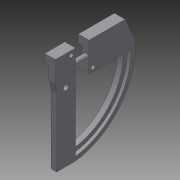
# Autodesk Inventor part: eye_cam_angled_bracket
Saved by Autodesk Inventor 2015 (Build 190159000, 159)
## iProperties
Created: 2015-06-20
Part Number: eye_cam_angled_bracket
Material: Generic
Document SubType Name: Modeling
Designer: Master
Density: 1 g/cm^3
Appearance: Default
Author: Master
Autodesk Inventor part; units mm, degrees
ref_plane "YZ Plane" through (0, 0, 0) normal (1, 0, 0) x (0, 1, 0)
ref_plane "XZ Plane" through (0, 0, 0) normal (0, 1, 0) x (-1, 0, 0)
ref_plane "XY Plane" through (0, 0, 0) normal (0, 0, 1) x (1, 0, 0)
sketch "Sketch1" plane through (0, 0, 0) normal (0, 0, 1) x (1, 0, 0)
  circle A0 centre (0, 0) radius 2
  dimension "d0" = 4
  constraints: 1 centre point, 1 coincident
  measures "d0" diameter of A0
extrude "Extrusion1" add sketch "Sketch1" against normal blind 40
sketch "Sketch2" plane through (0, 0, 0) normal (0, 0, 1) x (1, 0, 0)
  circle A0 centre (0, 0) radius 2 projected
  line L0 (2, -4.5) -> (-3, -4.5)
  line L1 (-3, -4.5) -> (-3, 4.5)
  line L2 (-3, 4.5) -> (2, 4.5)
  line L3 (2, 4.5) -> (2, -4.5)
  dimension "d3" = 3
  dimension "d4" = 9
  dimension "d5" = 4.5
  constraints: 8 end point, 1 tangent
  measures "d3" distance from line of L1 point (0, 0)
  measures "d4" distance between parallel lines of L2 L0
  measures "d5" distance from line of point (0, 0) L0
extrude "Extrusion2" add sketch "Sketch2" along normal blind 6 contours A0 | L3 L0 L1 L2
sketch "Sketch3" plane through (0, 0, 6) normal (0, 0, 1) x (1, 0, 0)
  circle A0 centre (0, 0) radius 2 projected
  line L0 (-3, -4.5) -> (2, -4.5) projected
  line L1 (2, -4.5) -> (2, 4.5) projected
  line L2 (2, 4.5) -> (-3, 4.5) projected
  line L3 (-3, 4.5) -> (-3, -4.5) projected
  line L4 (2, -4.5) -> (2, 4.5) projected
  line L5 (-3, 4.5) -> (2, 4.5)
  line L6 (2, 4.5) -> (2, 3.5)
  line L7 (2, 3.5) -> (-3, 3.5)
  line L8 (-3, 3.5) -> (-3, 4.5)
  point P0 (2, 0)
  dimension "d8" = 1
  constraints: 8 end point, 1 horizontal alignment, 1 point on line
  measures "d8" distance between parallel lines of L2 L7
extrude "Extrusion3" cut sketch "Sketch3" against normal blind 6 contours L7 L3 L2 L1
sketch "Sketch4" plane through (0, 0, -40) normal (0, 0, -1) x (-1, 0, 0)
  circle A0 centre (0, 0) radius 2 projected
extrude "Extrusion4" cut sketch "Sketch4" against normal blind 6
sketch "Sketch5" plane through (0, 0, -34) normal (0, 0, -1) x (-1, 0, 0)
  line L0 (3, 3.5) -> (-2, 3.5) projected
  line L1 (3, -4.5) -> (3, 3.5) projected
  line L2 (-2, 3.5) -> (-2, 0) projected
  line L3 (-2, 0) -> (-2, -4.5) projected
  line L4 (-2, -4.5) -> (3, -4.5) projected
  line L5 (3, 3.5) -> (-2, 3.5)
  line L6 (-2, 3.5) -> (-2, -4.5)
  line L7 (-2, -4.5) -> (3, -4.5)
  line L8 (3, -4.5) -> (3, 3.5)
  point P0 (0, 0)
  constraints: 8 end point
extrude "Extrusion5" add sketch "Sketch5" along normal blind 12
sketch "Sketch6" plane through (-3, -4.5, -34) normal (0, -1, 0) x (1, 0, 0)
  line L0 (5, 0) -> (0, 0) projected
  line L1 (0, 0) -> (0, -12) projected
  line L2 (5, -12) -> (0, -12) projected
  line L3 (5, 0) -> (5, -12) projected
  line L4 (5, -12) -> (0, -12)
  line L5 (0, -12) -> (0, 0)
  line L6 (0, 0) -> (5, 0)
  line L7 (5, 0) -> (5, -12)
  point P0 (3, 34)
  constraints: 8 end point
extrude "Extrusion6" add sketch "Sketch6" along normal blind 110
sketch "Sketch7" plane through (2, 0, -34) normal (1, 0, 0) x (0, 0, -1)
  line L0 (0, 3.5) -> (0, 0) projected
  line L1 (0, 0) -> (0, -114.5) projected
  line L2 (12, -114.5) -> (0, -114.5) projected
  line L3 (12, 3.5) -> (12, -114.5) projected
  line L4 (0, 3.5) -> (12, 3.5) projected
  line L5 (-34, 3.5) -> (-40, 3.5) projected
  line L6 (-40, -4.5) -> (-40, 3.5) projected
  line L7 (-34, -4.5) -> (-40, -4.5) projected
  line L8 (-34, 0) -> (-34, -4.5) projected
  line L9 (-34, 3.5) -> (-34, 0) projected
  line L10 (0, 3.5) -> (0, -114.5) projected
  line L11 (0, -108.5) -> (-25, -108.5)
  line L12 (-25, -108.5) -> (-25, -114.5)
  line L13 (-25, -114.5) -> (0, -114.5)
  line L14 (0, -114.5) -> (0, -108.5)
  line L15 (0, -114.5) -> (12, -114.5) projected
  line L16 (-40, -4.5) -> (-25, -108.5)
  line L17 (-34, -4.5) -> (-19, -108.5)
  point P0 (-34, 0)
  dimension "d46" = 6
  dimension "d47" = 25
  constraints: 12 end point, 2 point on line, 1 collinear, 1 parallel
  measures "d46" distance between parallel lines of L13 L11
  measures "d47" distance between parallel lines of L1 L12
extrude "Extrusion7" add sketch "Sketch7" against normal up to surface (5 mm away) contours L1 L13 L12 L11 | L11 L16 L7 L17 | L7 L6 L5 L9 L8
sketch "Sketch8" plane through (2, 3.5, 6) normal (1, 0, 0) x (0, 0, -1)
  line L0 (6, 0) -> (0, 0) projected
  line L1 (45, -10) -> (47, -10)
  line L2 (47, -10) -> (47, -112)
  line L3 (47, -112) -> (45, -112)
  line L4 (45, -112) -> (45, -10)
  line L5 (0, -8) -> (0, 0) projected
  line L6 (6, -3.5) -> (6, -8) projected
  line L7 (6, 0) -> (6, -3.5) projected
  line L8 (0, -8) -> (15, -112) projected
  line L9 (15, -112) -> (15, -118) projected
  line L10 (52, -118) -> (15, -118) projected
  line L11 (52, 0) -> (52, -118) projected
  line L12 (40, 0) -> (52, 0) projected
  line L13 (40, 0) -> (40, -3.5) projected
  line L14 (40, -3.5) -> (40, -112) projected
  line L15 (40, -112) -> (21, -112) projected
  line L16 (21, -112) -> (6, -8) projected
  dimension "d20" = 2
  dimension "d48" = 6
  dimension "d49" = 5
  dimension "d50" = 10
  constraints: 8 end point, 1 horizontal, 1 horizontal alignment
  measures "d20" distance between parallel lines of L4 L2
  measures "d48" distance from line of L10 L3.end
  measures "d49" distance between parallel lines of L11 L2
  measures "d50" distance between parallel lines of L1 L12
extrude "Extrusion8" cut sketch "Sketch8" against normal through all contours L1 L2 L3 L4
sketch "Sketch9" plane through (-3, 3.5, 0) normal (-1, 0, 0) x (0, 0, 1)
  line L0 (6, 0) -> (0, 0) projected
  line L1 (-46, 0) -> (-46, -118) projected
  line L2 (-46, -8) -> (-46, -9)
  line L3 (-34, -3.5) -> (-34, -112) projected
  line L4 (-34, -8) -> (-34, -9)
  line L5 (0, -8) -> (-0.8495, -13.8902)
  line L6 (-46, -9) -> (-34, -9)
  line L7 (6, -8) -> (0, -8)
  line L8 (-34, -8) -> (-46, -8)
  line L9 (0, -8) -> (0, 0) projected
  line L10 (6, 0) -> (6, -8) projected
  line L11 (-15, -112) -> (0, -8) projected
  line L12 (-34, -112) -> (-15, -112) projected
  line L13 (-34, 0) -> (-34, -112) projected
  line L14 (-34, 0) -> (-46, 0) projected
  line L15 (-46, 0) -> (-46, -118) projected
  line L16 (-9, -118) -> (-46, -118) projected
  line L17 (-9, -112) -> (-9, -118) projected
  line L18 (6, -8) -> (-9, -112) projected
  line L19 (-15, -112) -> (0, -8) projected
  line L20 (6, -8) -> (5.1505, -13.8902)
  line L21 (6, -8) -> (-9, -112) projected
  line L22 (5.1505, -13.8902) -> (-0.8495, -13.8902)
  line L23 (-15, -112) -> (0, -8) projected
  line L24 (-46, -9) -> (-34, -9)
  line L25 (-34, -9) -> (-34, -18.1174)
  line L26 (-34, -18.1174) -> (-46, -18.1174)
  line L27 (-46, -18.1174) -> (-46, -9)
  line L28 (-41, -9) -> (-41, -18.1174)
  line L29 (-41, -10) -> (-41, -112) projected
  line L30 (-39, -10) -> (-39, -112) projected
  line L31 (-39, -18.1174) -> (-39, -9)
  line L32 (-39, -10) -> (-39, -112) projected
  line L33 (-39, -112) -> (-41, -112) projected
  line L34 (-41, -112) -> (-41, -10) projected
  line L35 (-41, -10) -> (-39, -10) projected
  point P0 (0, -3.5)
  point P1 (-40, -8)
  point P2 (-39, 0)
  point P3 (-41, 0)
  constraints: 28 end point, 12 point on line, 1 collinear, 1 horizontal, 1 horizontal alignment, 1 midpoint
extrude "Extrusion9" add sketch "Sketch9" along normal blind 3.5 contours L18 L22 L5 L7 | L26 L30 L31 L6 L3 | L1 L6 L28 L26 | L6 L1 L8 L3
sketch "Sketch10" plane through (-3, 3.5, 6) normal (0, 1, 0) x (1, 0, 0)
  line L0 (2.5037, 5.3678) -> (4.55, 1.815)
  line L1 (4.55, 1.815) -> (2.4963, 0.6322)
  line L2 (2.4963, 0.6322) -> (0.45, 4.185)
  line L3 (0.45, 4.185) -> (2.5037, 5.3678)
  line L4 (0.45, 4.185) -> (4.55, 4.185)
  line L5 (4.55, 4.185) -> (4.55, 1.815)
  line L6 (4.55, 1.815) -> (0.45, 1.815)
  line L7 (0.45, 1.815) -> (0.45, 4.185)
  line L8 (2.5037, 5.3678) -> (4.55, 4.185)
  line L9 (0.45, 1.815) -> (2.4963, 0.6322)
  line L10 (2.4963, 45.3678) -> (4.5537, 41.8214)
  line L11 (4.5537, 41.8214) -> (2.5037, 40.6322)
  line L12 (2.5037, 40.6322) -> (0.4463, 44.1786)
  line L13 (0.4463, 44.1786) -> (2.4963, 45.3678)
  line L14 (0.4463, 44.1786) -> (4.5463, 44.1914)
  line L15 (4.5463, 44.1914) -> (4.5537, 41.8214)
  line L16 (4.5537, 41.8214) -> (0.4537, 41.8086)
  line L17 (0.4537, 41.8086) -> (0.4463, 44.1786)
  line L18 (2.4963, 45.3678) -> (4.5463, 44.1914)
  line L19 (0.4537, 41.8086) -> (2.5037, 40.6322)
  line L20 (4.4304, 1.8841) -> (2.4963, 0.6322)
  line L21 (0.4537, 41.8086) -> (4.5463, 44.1914)
  line L22 (4.5537, 41.8214) -> (0.4463, 44.1786)
  line L23 (2.5037, 40.6322) -> (2.4963, 45.3678)
  line L24 (5, 0) -> (0, 0) projected
  line L25 (0, 0) -> (0, 6) projected
  line L26 (0, 40) -> (5, 40) projected
  line L27 (0, 40) -> (0, 52) projected
  point P0 (3, 6)
  point P1 (11, 0)
  point P2 (11, 0)
  point P3 (2.5, 43)
  point P4 (2.5, 3)
  dimension "d28" = 4.1
  dimension "d29" = 2.37
  dimension "d30" = 4.1
  dimension "d31" = 2.37
  dimension "d33" = 4.1
  dimension "d34" = 2.37
  dimension "d35" = 4.1
  dimension "d36" = 2.37
  dimension "d38" = 3
  dimension "d39" = 2.5
  dimension "d40" = 3
  dimension "d41" = 2.5
  constraints: 48 end point, 2 perpendicular, 1 midpoint, 1 vertical alignment
  measures "d28" distance between parallel lines of L1 L3
  measures "d29" distance between parallel lines of L0 L2
  measures "d30" distance between parallel lines of L5 L7
  measures "d31" distance between parallel lines of L6 L4
  measures "d33" distance between parallel lines of L11 L13
  measures "d34" distance between parallel lines of L10 L12
  measures "d35" distance between parallel lines of L15 L17
  measures "d36" distance between parallel lines of L16 L14
  measures "d38" distance from line of point (2.5, 3) L24
  measures "d39" distance from line of point (2.5, 3) L25
  measures "d40" distance from line of L26 point (2.5, 43)
  measures "d41" distance from line of point (2.5, 43) L27
sketch "Sketch11" plane through (-3, 3.5, -34) normal (0, 1, 0) x (1, 0, 0)
  line L0 (0, 0) -> (5, 0) projected
  line L1 (5, 0) -> (5, 12) projected
  line L2 (0, 12) -> (5, 12) projected
  line L3 (0, 0) -> (0, 12) projected
  line L4 (5, -40) -> (0, -40) projected
  line L5 (5, -34) -> (5, -40) projected
  line L6 (0, -34) -> (5, -34) projected
  line L7 (0, -40) -> (0, -34) projected
  point P0 (3, -34)
extrude "Extrusion12" add sketch "Sketch11" along normal blind 2
sketch "Sketch12" plane through (2, -114.5, -9) normal (1, 0, 0) x (0, 0, -1)
  line L0 (30, 6) -> (30, 108) projected
  line L1 (30, 108) -> (32, 108) projected
  line L2 (32, 108) -> (32, 6) projected
  line L3 (32, 6) -> (30, 6) projected
  line L4 (-15, 110) -> (-15, 120) projected
  line L5 (-15, 110) -> (0, 6) projected
  line L6 (0, 6) -> (0, 0) projected
  line L7 (37, 0) -> (0, 0) projected
  line L8 (37, 0) -> (37, 120) projected
  line L9 (25, 120) -> (37, 120) projected
  line L10 (25, 114.5) -> (25, 120) projected
  line L11 (25, 114.5) -> (25, 6) projected
  line L12 (25, 6) -> (6, 6) projected
  line L13 (6, 6) -> (-9, 110) projected
  line L14 (-9, 114.5) -> (-9, 110) projected
  line L15 (-9, 120) -> (-9, 114.5) projected
  line L16 (-15, 120) -> (-9, 120) projected
  line L17 (-15, 120) -> (-9, 120)
  line L18 (-9, 120) -> (-9, 126)
  line L19 (-9, 126) -> (-15, 126)
  line L20 (-15, 126) -> (-15, 120)
  line L21 (25, 120) -> (37, 120)
  line L22 (37, 120) -> (37, 126)
  line L23 (37, 126) -> (25, 126)
  line L24 (25, 126) -> (25, 120)
  dimension "d53" = 6
  constraints: 16 end point, 1 point on line
  measures "d53" distance between parallel lines of L16 L19
extrude "Extrusion13" add sketch "Sketch12" against normal up to surface (8.5 mm away) contours L20 L19 L18 L16 | L9 L24 L23 L22
sketch "Sketch13" plane through (-6.5, 5.5, -46) normal (-1, 0, 0) x (0, 0, 1)
  line L0 (0, 0) -> (0, 6) projected
  line L1 (12, 0) -> (0, 0) projected
  line L2 (12, 6) -> (12, 0) projected
  line L3 (0, 6) -> (12, 6) projected
  line L4 (5, -11) -> (7, -11) projected
  line L5 (7, -11) -> (7, -20.1174) projected
  line L6 (7, -20.1174) -> (12, -20.1174) projected
  line L7 (12, -20.1174) -> (12, -10) projected
  line L8 (12, -10) -> (0, -10) projected
  line L9 (0, -10) -> (0, -20.1174) projected
  line L10 (0, -20.1174) -> (5, -20.1174) projected
  line L11 (5, -20.1174) -> (5, -11) projected
  line L12 (52, -10) -> (46, -10) projected
  line L13 (46, -10) -> (45.1505, -15.8902) projected
  line L14 (45.1505, -15.8902) -> (51.1505, -15.8902) projected
  line L15 (51.1505, -15.8902) -> (52, -10) projected
  line L16 (46, 0) -> (46, 6) projected
  line L17 (52, 0) -> (46, 0) projected
  line L18 (52, 6) -> (52, 0) projected
  line L19 (46, 6) -> (52, 6) projected
  point P0 (46, -5.5)
extrude "Extrusion14" cut sketch "Sketch13" against normal blind 0.5
sketch "Sketch14" plane through (0, 0, -34) normal (0, 0, 1) x (1, 0, 0)
  line L0 (-6, 11.5) -> (-6, 5.5) projected
  line L1 (-3, 5.5) -> (-6, 5.5) projected
  line L2 (-3, 5.5) -> (-3, -4.5) projected
  line L3 (-3, -4.5) -> (-6, -4.5) projected
  line L4 (-6, -4.5) -> (-6, -14.6174) projected
  line L5 (-3, -14.6174) -> (-6, -14.6174) projected
  line L6 (-3, -14.6174) -> (-3, -108.5) projected
  line L7 (-3, -108.5) -> (2, -108.5) projected
  line L8 (2, 0) -> (2, -108.5) projected
  circle A0 centre (0, 0) radius 2 projected
  line L9 (2, 0) -> (2, 11.5) projected
  line L10 (2, 11.5) -> (-6, 11.5) projected
  line L11 (2, 0) -> (2, 11.5) projected
  line L12 (-6, 11.5) -> (2, 11.5)
  line L13 (2, 11.5) -> (2, 5.5)
  line L14 (2, 5.5) -> (-6, 5.5)
  line L15 (-6, 5.5) -> (-6, 11.5)
  line L16 (2, 5.5) -> (-3, 5.5)
  line L17 (-3, 5.5) -> (-3, -4.5)
  line L18 (-3, -4.5) -> (2, -4.5)
  line L19 (2, -4.5) -> (2, 5.5)
  line L20 (-6, -14.6174) -> (2, -14.6174)
  line L21 (2, -14.6174) -> (2, -4.5)
  line L22 (2, -4.5) -> (-6, -4.5)
  line L23 (-6, -4.5) -> (-6, -14.6174)
  constraints: 24 end point, 1 horizontal alignment, 1 point on line
extrude "Extrusion15" add sketch "Sketch14" along normal blind 15 contours L10 L9 L14 L1 L0 | A0 | L14 L9 L8 L18 L2 | L18 L8 L20 L5 L4 L3
sketch "Sketch15" plane through (0, 0, 0) normal (0, 0, -1) x (-1, 0, 0)
  line L0 (6, 5.5) -> (6, 11.5) projected
  line L1 (-2, 11.5) -> (6, 11.5) projected
  line L2 (-2, 11.5) -> (-2, 0) projected
  circle A0 centre (0, 0) radius 2 projected
  line L3 (-2, 0) -> (-2, -4.5) projected
  line L4 (-2, -4.5) -> (3, -4.5) projected
  line L5 (3, -4.5) -> (3, 5.5) projected
  line L6 (3, 5.5) -> (6, 5.5) projected
  line L7 (6, -10.3902) -> (6, -4.5) projected
  line L8 (3, -4.5) -> (6, -4.5) projected
  line L9 (-2, -4.5) -> (3, -4.5) projected
  line L10 (-2, -108.5) -> (-2, -4.5) projected
  line L11 (3, -108.5) -> (-2, -108.5) projected
  line L12 (3, -108.5) -> (3, -10.3902) projected
  line L13 (3, -10.3902) -> (6, -10.3902) projected
  line L14 (-2, 11.5) -> (-2, 0) projected
  line L15 (6, 11.5) -> (-2, 11.5)
  line L16 (-2, 11.5) -> (-2, 5.5)
  line L17 (-2, 5.5) -> (6, 5.5)
  line L18 (6, 5.5) -> (6, 11.5)
  line L19 (-2, 5.5) -> (3, 5.5)
  line L20 (3, 5.5) -> (3, -4.5)
  line L21 (3, -4.5) -> (-2, -4.5)
  line L22 (-2, -4.5) -> (-2, 5.5)
  line L23 (6, -10.3902) -> (-2, -10.3902)
  line L24 (-2, -10.3902) -> (-2, -4.5)
  line L25 (-2, -4.5) -> (6, -4.5)
  line L26 (6, -4.5) -> (6, -10.3902)
  constraints: 24 end point, 1 horizontal alignment, 1 point on line
extrude "Extrusion16" add sketch "Sketch15" along normal blind 9 contours L6 L17 L2 L1 L0 | A0 | L5 L4 L3 L2 L17 | L8 L7 L13 L23 L10 L4
sketch "Sketch16" plane through (-3, -14.6174, -39) normal (0, -1, 0) x (1, 0, 0)
  line L0 (-3, 20) -> (-3, 0) projected
  line L1 (0, 0) -> (-3, 0) projected
  line L2 (0, 5) -> (0, 0) projected
  line L3 (5, 5) -> (0, 5) projected
  line L4 (5, 5) -> (5, 20) projected
  line L5 (-3, 20) -> (5, 20) projected
  line L6 (-3, -2) -> (-3, -7) projected
  line L7 (0, -7) -> (-3, -7) projected
  line L8 (0, -2) -> (0, -7) projected
  line L9 (0, -2) -> (-3, -2) projected
  point P0 (3, 39)
extrude "Extrusion17" cut sketch "Sketch16" against normal up to surface (4.2273 mm away)
sketch "Sketch17" plane through (-6, 5.5, -46) normal (-1, 0, 0) x (0, 0, 1)
  line L0 (0, -15.8902) -> (5, -15.8902) projected
  line L1 (5, -11) -> (5, -15.8902) projected
  line L2 (7, -11) -> (5, -11) projected
  line L3 (7, -15.8902) -> (7, -11) projected
  line L4 (7, -15.8902) -> (27, -15.8902) projected
  line L5 (27, -10) -> (27, -15.8902) projected
  line L6 (0, -10) -> (27, -10) projected
  line L7 (0, -15.8902) -> (0, -10) projected
  line L8 (5, -11) -> (7, -11)
  line L9 (7, -11) -> (7, -15.8902)
  line L10 (7, -15.8902) -> (5, -15.8902)
  line L11 (5, -15.8902) -> (5, -11)
  point P0 (46, -5.5)
  constraints: 8 end point
extrude "Extrusion18" add sketch "Sketch17" against normal up to surface (8 mm away) contours L1 L2 L3 L10
sketch "Sketch18" plane through (-6, 5.5, -46) normal (-1, 0, 0) x (0, 0, 1)
  line L0 (38.9361, 5) -> (42.4857, 2.9481)
  line L1 (42.4857, 2.9481) -> (41.2996, 0.8963)
  line L2 (41.2996, 0.8963) -> (37.75, 2.9481)
  line L3 (37.75, 2.9481) -> (38.9361, 5)
  line L4 (37.75, 2.9481) -> (41.2996, 5)
  line L5 (41.2996, 5) -> (42.4857, 2.9481)
  line L6 (42.4857, 2.9481) -> (38.9361, 0.8963)
  line L7 (38.9361, 0.8963) -> (37.75, 2.9481)
  line L8 (38.9361, 5) -> (41.2996, 5)
  line L9 (38.9361, 0.8963) -> (41.2996, 0.8963)
  line L10 (52, 0) -> (37, 0) projected
  line L11 (52, 6) -> (52, 0) projected
  line L12 (37, 6) -> (52, 6) projected
  line L13 (37, 0) -> (37, 6) projected
  line L14 (0, 0) -> (0, 6) projected
  line L15 (27, 0) -> (0, 0) projected
  line L16 (27, 6) -> (27, 0) projected
  line L17 (0, 6) -> (27, 6) projected
  line L18 (37, 6) -> (52, 6) projected
  line L19 (0, 6) -> (27, 6) projected
  line L20 (22.7004, 5) -> (26.25, 2.9481)
  line L21 (26.25, 2.9481) -> (25.0639, 0.8963)
  line L22 (25.0639, 0.8963) -> (21.5143, 2.9481)
  line L23 (21.5143, 2.9481) -> (22.7004, 5)
  line L24 (21.5143, 2.9481) -> (25.0639, 5)
  line L25 (25.0639, 5) -> (26.25, 2.9481)
  line L26 (26.25, 2.9481) -> (22.7004, 0.8963)
  line L27 (22.7004, 0.8963) -> (21.5143, 2.9481)
  line L28 (22.7004, 5) -> (25.0639, 5)
  line L29 (22.7004, 0.8963) -> (25.0639, 0.8963)
  line L30 (38.9361, -10.7865) -> (42.4857, -12.8383)
  line L31 (42.4857, -12.8383) -> (41.2996, -14.8902)
  line L32 (41.2996, -14.8902) -> (37.75, -12.8383)
  line L33 (37.75, -12.8383) -> (38.9361, -10.7865)
  line L34 (37.75, -12.8383) -> (41.2996, -10.7865)
  line L35 (41.2996, -10.7865) -> (42.4857, -12.8383)
  line L36 (42.4857, -12.8383) -> (38.9361, -14.8902)
  line L37 (38.9361, -14.8902) -> (37.75, -12.8383)
  line L38 (38.9361, -10.7865) -> (41.2996, -10.7865)
  line L39 (38.9361, -14.8902) -> (41.2996, -14.8902)
  line L40 (22.7004, -10.7865) -> (26.25, -12.8383)
  line L41 (26.25, -12.8383) -> (25.0639, -14.8902)
  line L42 (25.0639, -14.8902) -> (21.5143, -12.8383)
  line L43 (21.5143, -12.8383) -> (22.7004, -10.7865)
  line L44 (21.5143, -12.8383) -> (25.0639, -10.7865)
  line L45 (25.0639, -10.7865) -> (26.25, -12.8383)
  line L46 (26.25, -12.8383) -> (22.7004, -14.8902)
  line L47 (22.7004, -14.8902) -> (21.5143, -12.8383)
  line L48 (22.7004, -10.7865) -> (25.0639, -10.7865)
  line L49 (22.7004, -14.8902) -> (25.0639, -14.8902)
  line L50 (0, -15.8902) -> (27, -15.8902) projected
  line L51 (27, -10) -> (27, -15.8902) projected
  line L52 (0, -10) -> (27, -10) projected
  line L53 (0, -15.8902) -> (0, -10) projected
  line L54 (51.1505, -15.8902) -> (37, -15.8902) projected
  line L55 (52, -10) -> (51.1505, -15.8902) projected
  line L56 (37, -10) -> (52, -10) projected
  line L57 (37, -15.8902) -> (37, -10) projected
  line L58 (0, -15.8902) -> (27, -15.8902) projected
  line L59 (51.1505, -15.8902) -> (37, -15.8902) projected
  dimension "d66" = 4.1
  dimension "d67" = 2.37
  dimension "d68" = 4.1
  dimension "d69" = 2.37
  dimension "d79" = 0.75
  dimension "d80" = 1
  dimension "d81" = 4.1
  dimension "d82" = 2.37
  dimension "d83" = 4.1
  dimension "d84" = 2.37
  dimension "d85" = 0.75
  dimension "d88" = 4.1
  dimension "d89" = 2.37
  dimension "d90" = 4.1
  dimension "d91" = 2.37
  dimension "d92" = 4.1
  dimension "d93" = 2.37
  dimension "d94" = 4.1
  dimension "d95" = 2.37
  dimension "d96" = 1
  constraints: 80 end point, 4 parallel, 4 perpendicular, 2 horizontal alignment, 2 vertical alignment
  measures "d66" distance between parallel lines of L1 L3
  measures "d67" distance between parallel lines of L0 L2
  measures "d68" distance between parallel lines of L5 L7
  measures "d69" distance between parallel lines of L6 L4
  measures "d79" distance from line of L13 L2.end
  measures "d80" distance between parallel lines of L12 L8
  measures "d81" distance between parallel lines of L21 L23
  measures "d82" distance between parallel lines of L20 L22
  measures "d83" distance between parallel lines of L25 L27
  measures "d84" distance between parallel lines of L26 L24
  measures "d85" distance from line of L16 L20.end
  measures "d88" distance between parallel lines of L31 L33
  measures "d89" distance between parallel lines of L30 L32
  measures "d90" distance between parallel lines of L35 L37
  measures "d91" distance between parallel lines of L36 L34
  measures "d92" distance between parallel lines of L41 L43
  measures "d93" distance between parallel lines of L40 L42
  measures "d94" distance between parallel lines of L45 L47
  measures "d95" distance between parallel lines of L46 L44
  measures "d96" distance between parallel lines of L54 L39
extrude "Extrusion19" [suppressed]
sketch "Sketch19" plane through (2, -108.5, -15) normal (1, 0, 0) x (0, 0, -1)
  line L0 (-6, 104) -> (-21, 104) projected
  line L1 (4, 98.1098) -> (19, 98.1098) projected
  line L2 (19, 98.1098) -> (19, 0) projected
  line L3 (19, 0) -> (0, 0) projected
  line L4 (0, 0) -> (-14.1505, 98.1098) projected
  line L5 (-14.1505, 98.1098) -> (-6, 98.1098) projected
  line L6 (-6, 108.5) -> (-6, 98.1098) projected
  line L7 (-6, 120) -> (-6, 108.5) projected
  line L8 (-6, 120) -> (-21, 120) projected
  line L9 (-21, 104) -> (-21, 120) projected
  line L10 (-21, 104) -> (-6, 0) projected
  line L11 (-6, 0) -> (-6, -6) projected
  line L12 (31, -6) -> (-6, -6) projected
  line L13 (31, -6) -> (31, 120) projected
  line L14 (31, 120) -> (4, 120) projected
  line L15 (4, 108.5) -> (4, 120) projected
  line L16 (4, 98.1098) -> (4, 108.5) projected
  line L17 (26, 98.1098) -> (24, 98.1098) projected
  line L18 (26, 98.1098) -> (26, 0) projected
  line L19 (26, 0) -> (24, 0) projected
  line L20 (24, 0) -> (24, 98.1098) projected
  line L21 (31, 98.1098) -> (-21, 98.1098)
  line L22 (-21, 98.1098) -> (-21, -6)
  line L23 (-21, -6) -> (31, -6)
  line L24 (31, -6) -> (31, 98.1098)
  point P0 (-15, 108.5)
  constraints: 8 end point
extrude "Extrusion20" cut sketch "Sketch19" against normal through all contours L21 L1 L2 L3 L4 L5 | L21 L4 L3 L2 L20 L19 L18 L13 L12 L11 L10 | L10 L11 L23 L22 L21
sketch "Sketch20" plane through (-6, -10.3902, 5.1505) normal (0, -1, 0) x (1, 0, 0)
  line L0 (0, 0) -> (8, 0) projected
  line L1 (0, 0) -> (0, -14.1505) projected
  line L2 (8, -14.1505) -> (0, -14.1505) projected
  line L3 (8, 0) -> (8, -14.1505) projected
  point P0 (6, -5.1505)
extrude "Extrusion21" add sketch "Sketch20" along normal blind 40
sketch "Sketch22" plane through (-6, 5.5, -46) normal (-1, 0, 0) x (0, 0, 1)
  line L0 (52, -10) -> (51.1505, -15.8902) projected
  line L1 (37, -10) -> (52, -10) projected
  line L2 (37, -10) -> (37, -55.8902) projected
  line L3 (51.1505, -55.8902) -> (37, -55.8902) projected
  line L4 (51.1505, -15.8902) -> (51.1505, -55.8902) projected
  line L5 (0, -15.8902) -> (27, -15.8902) projected
  line L6 (27, -10) -> (27, -15.8902) projected
  line L7 (0, -10) -> (27, -10) projected
  line L8 (0, -15.8902) -> (0, -10) projected
  line L9 (37, -10) -> (37, -55.8902) projected
  line L10 (37, -15.8902) -> (51.1505, -15.8902)
  line L11 (51.1505, -15.8902) -> (51.1505, -55.8902)
  line L12 (51.1505, -55.8902) -> (37, -55.8902)
  line L13 (37, -55.8902) -> (37, -15.8902)
  point P0 (46, -5.5)
  constraints: 8 end point, 1 point on line
extrude "Extrusion22" cut sketch "Sketch22" against normal blind 2 contours L4 L3 L2 L10
sketch "Sketch23" plane through (2, -4.5, 6) normal (1, 0, 0) x (0, 0, -1)
  line L0 (15, 4.5) -> (15, -45.8902) projected
  line L1 (15, 16) -> (15, 4.5) projected
  line L2 (15, 16) -> (0, 16) projected
  line L3 (0, 0) -> (0, 16) projected
  line L4 (0, 0) -> (0.8495, -5.8902) projected
  line L5 (0.8495, -5.8902) -> (0.8495, -45.8902) projected
  line L6 (15, -45.8902) -> (0.8495, -45.8902) projected
  line L7 (25, -5.8902) -> (52, -5.8902) projected
  line L8 (52, -5.8902) -> (52, 16) projected
  line L9 (52, 16) -> (25, 16) projected
  line L10 (25, 4.5) -> (25, 16) projected
  line L11 (25, -5.8902) -> (25, 4.5) projected
  line L12 (15, -5.8902) -> (0.8495, -5.8902) projected
  arc A0 (15, -49.3938) -> (52, -5.8902) centre (7.9248, -5.8902) ccw
  line L13 (15, -45.8902) -> (0.8495, -45.8902)
  line L14 (0.8495, -45.8902) -> (0.8495, -55.4631)
  line L15 (0.8495, -55.4631) -> (15, -55.4631)
  line L16 (15, -49.3938) -> (15, -45.8902)
  line L17 (58, -5.8902) -> (58, -1.9112)
  line L18 (58, -1.9112) -> (52, -1.9112)
  line L19 (52, -1.9112) -> (52, -5.8902)
  line L20 (15, -49.3938) -> (0.8495, -49.3938)
  line L21 (0.8495, -49.3938) -> (0.8495, -45.8902)
  line L22 (0.8495, -45.8902) -> (15, -45.8902)
  arc A1 (15, -55.4631) -> (58, -5.8902) centre (7.9248, -5.8902) ccw
  arc A2 (14.7799, -50.9469) -> (53.5, -5.8902) centre (7.9248, -5.8902) ccw
  arc A3 (14.9729, -53.9514) -> (56.5, -5.8902) centre (7.9248, -5.8902) ccw
  line L23 (52, -5.8902) -> (53.5, -5.8902)
  line L24 (56.5, -5.8902) -> (58, -5.8902)
  line L25 (15, -55.4631) -> (15, -53.9474)
  line L26 (15, -50.9129) -> (15, -49.3938)
  line L27 (53.5, -5.8902) -> (56.5, -5.8902)
  line L28 (15, -53.9474) -> (15, -50.9129)
  point P0 (6, 4.5)
  dimension "d104" = 6
  dimension "d105" = 3
  dimension "d106" = 1.5
  constraints: 33 end point, 10 point on circle, 4 centre point, 3 coincident, 1 midpoint
  measures "d104" distance of L7.end L17.start
  measures "d105" radial gap between concentric circles of A3 A2
  measures "d106" radial gap between concentric circles of A0 A2
extrude "Extrusion23" add sketch "Sketch23" against normal blind 4 contours L16 L20 L14 L6 | L26 L28 L25 L15 L14 L20 | A0 L23 A2 L26 | L8 L18 L17 L24 L27 L23 | A3 L24 A1 L25
sketch "Sketch24" plane through (2, -4.5, 6) normal (1, 0, 0) x (0, 0, -1)
  line L0 (15, -53.9474) -> (15, -50.9129) projected
  arc A0 (15, -50.9129) -> (53.5, -5.8902) centre (7.9248, -5.8902) ccw projected
  line L1 (53.5, -5.8902) -> (56.5, -5.8902) projected
  arc A1 (15, -53.9474) -> (56.5, -5.8902) centre (7.9248, -5.8902) ccw projected
  line L2 (15, 4.5) -> (15, -49.3938) projected
  line L3 (15, 16) -> (15, 4.5) projected
  line L4 (15, 16) -> (0, 16) projected
  line L5 (0, 0) -> (0, 16) projected
  line L6 (0, 0) -> (0.8495, -5.8902) projected
  line L7 (0.8495, -5.8902) -> (0.8495, -55.4631) projected
  line L8 (0.8495, -55.4631) -> (15, -55.4631) projected
  arc A2 (15, -55.4631) -> (58, -5.8902) centre (7.9248, -5.8902) ccw projected
  line L9 (58, -5.8902) -> (58, -1.9112) projected
  line L10 (58, -1.9112) -> (52, -1.9112) projected
  line L11 (52, -1.9112) -> (52, 16) projected
  line L12 (52, 16) -> (25, 16) projected
  line L13 (25, 4.5) -> (25, 16) projected
  line L14 (25, -5.8902) -> (25, 4.5) projected
  line L15 (25, -5.8902) -> (52, -5.8902) projected
  arc A3 (15, -49.3938) -> (52, -5.8902) centre (7.9248, -5.8902) ccw projected
  line L16 (25, -5.8902) -> (52, -5.8902) projected
  arc A4 (15, -47.8734) -> (50.5, -5.8902) centre (7.9248, -5.8902) ccw
  arc A5 (14.7221, -57.0155) -> (59.5, -5.8902) centre (7.9248, -5.8902) ccw
  line L17 (0.8495, -55.4631) -> (14.7221, -55.4631)
  line L18 (14.7221, -55.4631) -> (14.7221, -57.0155)
  line L19 (14.7221, -57.0155) -> (0.8495, -57.0155)
  line L20 (0.8495, -57.0155) -> (0.8495, -55.4631)
  line L21 (58, -5.8902) -> (59.5, -5.8902)
  line L22 (58, -1.9112) -> (59.5, -1.9112)
  line L23 (59.5, -1.9112) -> (59.5, -5.8902)
  line L24 (59.5, -5.8902) -> (58, -5.8902)
  line L25 (58, -5.8902) -> (58, -1.9112)
  point P0 (6, 4.5)
  dimension "d109" = 1.5
  dimension "d110" = 1.5
  constraints: 19 end point, 4 point on circle, 2 centre point, 2 coincident, 2 point on line
  measures "d109" radial gap between concentric circles of A3 A4
  measures "d110" radial gap between concentric circles of A2 A5
extrude "Extrusion24" add sketch "Sketch24" against normal blind 4 contours A4 L15 A3 L2 | L8 L18 L19 L20 | L8 A2 L21 A5 L18 | L22 L23 L21 L9
sketch "Sketch25" plane through (2, -4.5, 6) normal (1, 0, 0) x (0, 0, -1)
  line L0 (15, -53.9474) -> (15, -50.9129) projected
  arc A0 (15, -50.9129) -> (53.5, -5.8902) centre (7.9248, -5.8902) ccw projected
  line L1 (53.5, -5.8902) -> (56.5, -5.8902) projected
  arc A1 (15, -53.9474) -> (56.5, -5.8902) centre (7.9248, -5.8902) ccw projected
  line L2 (15, 4.5) -> (15, -47.8734) projected
  line L3 (15, 16) -> (15, 4.5) projected
  line L4 (15, 16) -> (0, 16) projected
  line L5 (0, 0) -> (0, 16) projected
  line L6 (0, 0) -> (0.8495, -5.8902) projected
  line L7 (0.8495, -5.8902) -> (0.8495, -57.0155) projected
  line L8 (0.8495, -57.0155) -> (14.7221, -57.0155) projected
  arc A2 (14.7221, -57.0155) -> (59.5, -5.8902) centre (7.9248, -5.8902) ccw projected
  line L9 (59.5, -5.8902) -> (59.5, -1.9112) projected
  line L10 (59.5, -1.9112) -> (52, -1.9112) projected
  line L11 (52, -1.9112) -> (52, 16) projected
  line L12 (52, 16) -> (25, 16) projected
  line L13 (25, 4.5) -> (25, 16) projected
  line L14 (25, -5.8902) -> (25, 4.5) projected
  line L15 (25, -5.8902) -> (50.5, -5.8902) projected
  arc A3 (15, -47.8734) -> (50.5, -5.8902) centre (7.9248, -5.8902) ccw projected
  line L16 (52, 16) -> (59.5, -1.9112)
  point P0 (6, 4.5)
  constraints: 2 end point
extrude "Extrusion25" add sketch "Sketch25" against normal blind 4 contours L16 L10 L11
sketch "Sketch26" plane through (-6, 5.5, -46) normal (-1, 0, 0) x (0, 0, 1)
  circle A0 centre (23.8821, 2.9481) radius 1.5
  circle A1 centre (23.8821, -12.8383) radius 1.5
  circle A2 centre (40.1179, 2.9481) radius 1.5
  circle A3 centre (40.1179, -12.8383) radius 1.5
  point P0 (46, -5.5)
  dimension "d115" = 3
  dimension "d116" = 3
  dimension "d117" = 3
  dimension "d118" = 3
  constraints: 4 centre point, 4 coincident
  measures "d115" diameter of A0
  measures "d116" diameter of A1
  measures "d117" diameter of A2
  measures "d118" diameter of A3
extrude "Extrusion26" cut sketch "Sketch26" against normal through all contours A1 | A2
sketch "Sketch27" plane through (2, -4.5, 6) normal (1, 0, 0) x (0, 0, -1)
  arc A0 (15, -47.8734) -> (50.5, -5.8902) centre (7.9248, -5.8902) ccw projected
  circle A1 centre (7.9248, -5.8902) radius 2
  point P0 (6, 4.5)
  dimension "d121" = 4
  constraints: 1 centre point, 1 coincident
  measures "d121" diameter of A1
extrude "Extrusion27" cut sketch "Sketch27" against normal through all
sketch "Sketch28" plane through (-6, 5.5, -46) normal (-1, 0, 0) x (0, 0, 1)
  arc A0 (46.0752, -15.8902) -> (42.0752, -15.8902) centre (44.0752, -15.8902) ccw projected
  line L0 (46.0752, -15.8902) -> (51.1505, -15.8902) projected
  line L1 (52, -10) -> (51.1505, -15.8902) projected
  line L2 (37, -10) -> (52, -10) projected
  line L3 (37, -10) -> (37, -15.8902) projected
  line L4 (37, -15.8902) -> (42.0752, -15.8902) projected
  line L5 (37, -15.8902) -> (42.0752, -15.8902) projected
  line L6 (40.5881, -15.8902) -> (52, -15.8902)
  line L7 (52, -15.8902) -> (52, -10)
  line L8 (52, -10) -> (40.5881, -10)
  line L9 (40.5881, -10) -> (40.5881, -15.8902)
  point P0 (46, -5.5)
  constraints: 8 end point, 1 point on line
extrude "Extrusion28" cut sketch "Sketch28" against normal up to surface (2 mm away) contours A0 L4 L9 L2 L1 L0
sketch "Sketch29" plane through (-4, 5.5, -46) normal (-1, 0, 0) x (0, 0, 1)
  line L0 (37, -15.8902) -> (40.5881, -15.8902) projected
  line L1 (37, -55.8902) -> (37, -15.8902) projected
  line L2 (51.1505, -55.8902) -> (37, -55.8902) projected
  line L3 (51.1505, -15.8902) -> (51.1505, -55.8902) projected
  line L4 (52, -10) -> (51.1505, -15.8902) projected
  line L5 (40.5881, -10) -> (52, -10) projected
  line L6 (40.5881, -10) -> (40.5881, -15.8902) projected
  circle A0 centre (44.0752, -15.8902) radius 2 projected
  line L7 (51.1505, -55.8902) -> (37, -55.8902)
  line L8 (37, -55.8902) -> (37, -15.8902)
  line L9 (37, -15.8902) -> (51.1505, -15.8902)
  line L10 (51.1505, -15.8902) -> (51.1505, -55.8902)
  point P0 (46, -5.5)
  constraints: 8 end point
extrude "Extrusion29" cut sketch "Sketch29" against normal up to surface (2 mm away) contours L0 L9 A0 L3 L2 L1 | L9 A0 picked at (43.9948, -16.552)
sketch "Sketch30" plane through (-6, 5.5, -46) normal (-1, 0, 0) x (0, 0, 1)
  line L0 (40.5881, -15.8902) -> (40.5881, -10) projected
  line L1 (37, -10) -> (40.5881, -10) projected
  line L2 (37, -10) -> (37, -15.8902) projected
  line L3 (37, -15.8902) -> (40.5881, -15.8902) projected
  line L4 (46.0752, -15.8902) -> (51.1505, -15.8902) projected
  line L5 (52, -10) -> (51.1505, -15.8902) projected
  line L6 (40.5881, -10) -> (52, -10) projected
  line L7 (40.5881, -10) -> (40.5881, -15.8902) projected
  line L8 (40.5881, -15.8902) -> (42.0752, -15.8902) projected
  arc A0 (46.0752, -15.8902) -> (42.0752, -15.8902) centre (44.0752, -15.8902) ccw projected
  line L9 (37, -10) -> (52, -10)
  line L10 (52, -10) -> (52, -15.8902)
  line L11 (52, -15.8902) -> (37, -15.8902)
  line L12 (37, -15.8902) -> (37, -10)
  point P0 (46, -5.5)
  constraints: 8 end point
extrude "Extrusion30" cut sketch "Sketch30" against normal up to surface (4 mm away)
sketch "Sketch31" plane through (-2, -4.5, 6) normal (-1, 0, 0) x (0, 0, 1)
  circle A0 centre (-7.9248, -5.8902) radius 2 projected
  arc A1 (-56.5, -5.8902) -> (-15, -53.9474) centre (-7.9248, -5.8902) ccw projected
  line L0 (-56.5, -5.8902) -> (-53.5, -5.8902) projected
  arc A2 (-53.5, -5.8902) -> (-15, -50.9129) centre (-7.9248, -5.8902) ccw projected
  line L1 (-15, -50.9129) -> (-15, -53.9474) projected
  line L2 (0, 0) -> (-0.8495, -5.8902) projected
  line L3 (-15, 0) -> (0, 0) projected
  line L4 (-15, -47.8734) -> (-15, 0) projected
  arc A3 (-50.5, -5.8902) -> (-15, -47.8734) centre (-7.9248, -5.8902) ccw projected
  line L5 (-52, -5.8902) -> (-50.5, -5.8902) projected
  line L6 (-52, 16) -> (-52, -5.8902) projected
  line L7 (-52, 16) -> (-59.5, -1.9112) projected
  line L8 (-59.5, -1.9112) -> (-59.5, -5.8902) projected
  arc A4 (-59.5, -5.8902) -> (-14.7221, -57.0155) centre (-7.9248, -5.8902) ccw projected
  line L9 (-14.7221, -57.0155) -> (-0.8495, -57.0155) projected
  line L10 (-0.8495, -5.8902) -> (-0.8495, -57.0155) projected
  circle A5 centre (-28.1179, -2.8383) radius 1.5 projected
  line L11 (-52, -5.8902) -> (-25, -5.8902) projected
  line L12 (-25, 0) -> (-25, -5.8902) projected
  line L13 (-52, 0) -> (-25, 0) projected
  line L14 (-52, -5.8902) -> (-52, 0) projected
  line L15 (-59.5, -5.8902) -> (-0.8495, -5.8902)
  line L16 (-0.8495, -5.8902) -> (-0.8495, -57.0155)
  line L17 (-0.8495, -57.0155) -> (-59.5, -57.0155)
  line L18 (-59.5, -57.0155) -> (-59.5, -5.8902)
  point P0 (-6, 4.5)
  constraints: 8 end point
extrude "Extrusion31" [suppressed]
equation "\"d5\" = 0.5 * d4"
body "Solid1"
